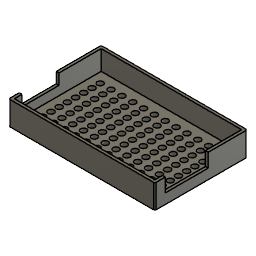
Screen_Cover (Autodesk Fusion 360 design; units mm, degrees)
part number: 2026-01-27-21-39-35-772
Autodesk Fusion 360 part; units mm, degrees
sketch "Esquisse1" plane through (0, 0, 0) normal (0, 1, 0) x (1, 0, 0)
  line L0 (117.75, 72.75) -> (-117.75, 72.75)
  line L1 (-117.75, 72.75) -> (-117.75, -72.75)
  line L2 (-117.75, -72.75) -> (117.75, -72.75)
  line L3 (117.75, -72.75) -> (117.75, 72.75)
  line L4 (117.75, 72.75) -> (-117.75, -72.75) construction
  line L5 (-117.75, 72.75) -> (117.75, -72.75) construction
  line L6 (122.5, 77.5) -> (-122.5, 77.5)
  line L7 (-122.5, 77.5) -> (-122.5, -77.5)
  line L8 (-122.5, -77.5) -> (122.5, -77.5)
  line L9 (122.5, -77.5) -> (122.5, 77.5)
  line L10 (122.5, 77.5) -> (-122.5, -77.5) construction
  line L11 (-122.5, 77.5) -> (122.5, -77.5) construction
  dimension "d4" = 145.5
  dimension "d5" = 235.5
  dimension "d6" = 155
  dimension "d7" = 245
  constraint horizontal L0
  constraint perpendicular L0 L1
  constraint parallel L0 L2
  constraint parallel L1 L3
  constraint coincident L4 origin
  constraint coincident L5 origin
  constraint horizontal L6
  constraint perpendicular L6 L7
  constraint parallel L6 L8
  constraint parallel L7 L9
  constraint coincident L10 origin
  constraint coincident L11 origin
  measures "d4" distance of L0.end L1.end
  measures "d5" distance of L0.start L0.end
  measures "d6" distance of L6.start L8.end
  measures "d7" distance of L7.end L8.end
extrude "Extrusion1" add sketch "Esquisse1" along normal blind 40
extrude "Extrusion2" add sketch "Esquisse1" along normal blind 7 contours L0 L1 L2 L3
sketch "Esquisse3" plane through (122.5, 0, 0) normal (1, 0, 0) x (0, 0, -1)
  line L0 (-77.5, 0) -> (77.5, 0)
  line L1 (77.5, 0) -> (77.5, 40)
  line L2 (77.5, 40) -> (-77.5, 40)
  line L3 (-77.5, 40) -> (-77.5, 0)
  line L4 (-60, 40) -> (2, 40)
  line L5 (2, 40) -> (2, 17)
  line L6 (2, 17) -> (-60, 17)
  line L7 (-60, 17) -> (-60, 40)
  dimension "d24" = 62
  dimension "d25" = 23
  dimension "d26" = 17.5
  dimension "d28" = 23
  constraint horizontal L4
  constraint vertical L5
  constraint horizontal L6
  constraint vertical L7
  measures "d24" distance of L4.start L4.end
  measures "d25" distance of L4.start L6.end
  measures "d26" distance of L3 L7
  measures "d28" distance of L2 L6
extrude "Extrusion5" cut sketch "Esquisse3" against normal blind 260 contours L2 L4 L5 L6 L7
extrude "Extrusion6" add 1 faces at (-119.3333, 17, 18.6667) along direction (0, 1, 0) blind 5
fillet "Congé1" radius 2 4 edges at (122.5, 20, -77.5) (122.5, 20, 77.5) (-122.5, 20, 77.5) (-122.5, 20, -77.5)
hole "Perçage1" at (98.8567, 7, -54.5653) direction (0, -1, 0) diameter 10 depth 10 tip angle 118
pattern_linear "Réseau R1" count 12 spacing 18.1818 along (-1, 0, 0) count 9 spacing 13.75 along (0, 0, 1) of "Perçage1"
extrude "Extrusion7" cut 1 faces at (120.9167, 32.3333, -2) along direction (0, 0, -1) blind 10
